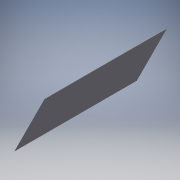
# Autodesk Inventor part: Seitenteil_Einbau2
Saved by Autodesk Inventor 2016 (Build 200138000, 138)
## iProperties
Created: 2017-04-21
Part Number: Seitenteil_Einbau2
Material: Generic
Document SubType Name: Modeling
Designer: reinert
Density: 1 g/cm^3
Appearance: Default
Author: reinert
Autodesk Inventor part; units mm, degrees
ref_plane "YZ Plane" through (0, 0, 0) normal (1, 0, 0) x (0, 1, 0)
ref_plane "XZ Plane" through (0, 0, 0) normal (0, 1, 0) x (-1, 0, 0)
ref_plane "XY Plane" through (0, 0, 0) normal (0, 0, 1) x (1, 0, 0)
sketch "Sketch1" plane through (0, 0, 0) normal (0, 0, 1) x (1, 0, 0)
  line L0 (0, 0) -> (-2, 0)
  line L1 (-2, 0) -> (-2, 540)
  line L2 (-2, 540) -> (0, 540)
  line L3 (0, 540) -> (0, 0)
  dimension "d0" = 2
  dimension "d1" = 540
  constraints: 8 end point, 2 parallel, 1 horizontal, 1 perpendicular
  measures "d0" distance of L0.start L0.end
  measures "d1" distance of L0.end L1.end
extrude "Extrusion1" add sketch "Sketch1" along normal blind 90
body "Solid1"
